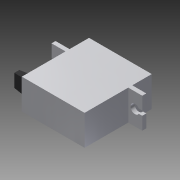
# Autodesk Inventor part: serwo HK15148
Saved by Autodesk Inventor 2013 (Build 170138000, 138)
## iProperties
Created: 2013-03-06
Part Number: serwo HK15148
Material: Generic
Document SubType Name: Modeling
Designer: Masta
Density: 1 g/cm^3
Author: Masta
Autodesk Inventor part; units mm, degrees
ref_plane "YZ Plane" through (0, 0, 0) normal (1, 0, 0) x (0, 1, 0)
ref_plane "XZ Plane" through (0, 0, 0) normal (0, 1, 0) x (-1, 0, 0)
ref_plane "XY Plane" through (0, 0, 0) normal (0, 0, 1) x (1, 0, 0)
sketch "Sketch1" plane through (0, 0, 0) normal (0, 1, 0) x (-1, 0, 0)
  line L0 (14, 6.75) -> (-14, 6.75)
  line L1 (-14, 6.75) -> (-14, -6.75)
  line L2 (-14, -6.75) -> (14, -6.75)
  line L3 (14, -6.75) -> (14, 6.75)
  line L4 (14, 6.75) -> (-14, -6.75) construction
  line L5 (-14, 6.75) -> (14, -6.75) construction
  line L6 (20.25, -6.75) -> (20.25, -1)
  line L7 (14, -6.75) -> (20.25, -6.75)
  line L8 (14, 6.75) -> (20.25, 6.75)
  line L9 (-14, 6.75) -> (-20.25, 6.75)
  line L10 (-14, -6.75) -> (-20.25, -6.75)
  line L11 (-14, 0) -> (14, 0) construction
  line L12 (0, 6.75) -> (0, -6.75) construction
  line L13 (20.25, -1) -> (18.7321, -1)
  line L14 (20.25, 1) -> (18.7321, 1)
  circle A0 centre (17, 0) radius 2
  line L15 (-20.25, 6.75) -> (-20.25, -6.75)
  line L16 (20.25, 1) -> (20.25, 6.75)
  line L17 (20.25, -1) -> (20.25, 1)
  line L18 (-20.25, 6.75) -> (20.25, -6.75) construction
  line L19 (-20.25, -6.75) -> (20.25, 6.75) construction
  line L20 (17, 0) -> (14, 0) construction
  point P0 (0, 0)
  point P1 (0, 0)
  dimension "d0" = 28
  dimension "d1" = 13.5
  dimension "d2" = 40.5
  dimension "d40" = 4
  dimension "d41" = 2
  dimension "d42" = 17
  constraints: 42 end point, 7 midpoint, 7 parallel, 5 perpendicular, 2 collinear, 2 point on circle, 1 centre point, 1 coincident, 1 horizontal, 1 other
  measures "d0" distance of L2.end L1.end
  measures "d1" distance of L1.end L0.end
  measures "d2" distance of L10.end L6.start
  measures "d40" diameter of A0
  measures "d41" distance between parallel lines of L14 L13
  measures "d42" distance of point (0, 0) L20.start
extrude "Extrusion1" add sketch "Sketch1" along normal blind 10.5 and the other way blind 19.5 contours L3 L2 L1 L0
extrude "Extrusion2" add sketch "Sketch1" along normal blind 1.8 contours L8 L16 L14 A0 L13 L6 L7 L3
sketch "Sketch2" plane through (0, 10.5, 0) normal (0, 1, 0) x (1, 0, 0)
  line L0 (-14, 6.75) -> (-14, -6.75) projected
  circle A0 centre (-4, 0) radius 6.5
  line L1 (-4, 0) -> (0, 0) construction
  dimension "d14" = 13
  dimension "d15" = 10
  constraints: 2 end point, 1 centre point, 1 perpendicular
  measures "d14" diameter of A0
  measures "d15" distance from line of L1.start L0
extrude "Extrusion3" add sketch "Sketch2" along normal blind 0.1
sketch "Sketch3" plane through (-4, 10.6, 0) normal (0, 1, 0) x (1, 0, 0)
  circle A0 centre (0, 0) radius 6.5 projected
  circle A1 centre (0, 0) radius 3
  point P0 (4, 0)
  dimension "d18" = 6
  constraints: 1 centre point, 1 coincident
  measures "d18" diameter of A1
extrude "Extrusion4" add sketch "Sketch3" along normal blind 3.5 contours A1
sketch "Sketch4" plane through (-14, -19.5, -6.75) normal (-1, 0, 0) x (0, 0, 1)
  line L0 (13.5, 19.5) -> (0, 19.5) projected
  line L1 (3.25, 3) -> (10.25, 3)
  line L2 (10.25, 3) -> (10.25, 6.5)
  line L3 (10.25, 6.5) -> (3.25, 6.5)
  line L4 (3.25, 6.5) -> (3.25, 3)
  line L5 (3.25, 3) -> (10.25, 6.5) construction
  line L6 (10.25, 3) -> (3.25, 6.5) construction
  line L7 (6.75, 19.5) -> (6.75, 4.75) construction
  dimension "d21" = 7
  dimension "d22" = 3.5
  dimension "d23" = 13
  constraints: 14 end point, 3 parallel, 2 midpoint, 1 horizontal, 1 perpendicular
  measures "d21" distance of L3.end L2.end
  measures "d22" distance of L2.end L1.end
  measures "d23" distance between parallel lines of L0 L3
extrude "Extrusion5" add sketch "Sketch4" along normal blind 7 draft -5
sketch "Sketch6" plane through (0, 10.5, 0) normal (0, 1, 0) x (1, 0, 0)
  line L0 (9.5237, -5.9702) -> (9.5237, 8.1574) construction
  line L1 (9.5237, 8.1574) -> (13.0974, 8.1574) construction
  line L2 (13.0974, 8.1574) -> (13.0974, -5.9702) construction
  line L3 (13.0974, -5.9702) -> (9.5237, -5.9702) construction
  line L4 (11.569, -4.3154) -> (11.569, -4.5812)
  line L5 (11.569, -4.5812) -> (10.5901, -4.5812)
  line L6 (10.5901, -4.5812) -> (10.5901, -5.5018)
  line L7 (10.5901, -5.5018) -> (11.569, -5.5018)
  line L8 (11.569, -5.5018) -> (11.569, -5.7676)
  line L9 (11.569, -5.7676) -> (9.569, -5.7676)
  line L10 (9.569, -5.7676) -> (9.569, -5.5018)
  line L11 (9.569, -5.5018) -> (10.3535, -5.5018)
  line L12 (10.3535, -5.5018) -> (10.3535, -4.5812)
  line L13 (10.3535, -4.5812) -> (9.569, -4.5812)
  line L14 (9.569, -4.5812) -> (9.569, -4.3154)
  line L15 (9.569, -4.3154) -> (11.569, -4.3154)
  line L16 (11.569, -2.4516) -> (11.569, -2.7968)
  line L17 (11.569, -2.7968) -> (10.6387, -3.5278)
  line L18 (10.6387, -3.5278) -> (10.77, -3.6445)
  line L19 (10.77, -3.6445) -> (11.569, -3.6445)
  line L20 (11.569, -3.6445) -> (11.569, -3.9103)
  line L21 (11.569, -3.9103) -> (9.569, -3.9103)
  line L22 (9.569, -3.9103) -> (9.569, -3.6445)
  line L23 (9.569, -3.6445) -> (10.488, -3.6445)
  line L24 (10.488, -3.6445) -> (9.569, -2.8244)
  line L25 (9.569, -2.8244) -> (9.569, -2.5002)
  line L26 (9.569, -2.5002) -> (10.4621, -3.3284)
  line L27 (10.4621, -3.3284) -> (11.569, -2.4516)
  line L28 (11.569, -1.2166) -> (11.569, -2.1923)
  line L29 (11.569, -2.1923) -> (11.3648, -2.1923)
  line L30 (11.3648, -2.1923) -> (11.3648, -1.8292)
  line L31 (11.3648, -1.8292) -> (10.0245, -1.8292)
  line L32 (10.0245, -1.8292) -> (10.0245, -2.1923)
  line L33 (10.0245, -2.1923) -> (9.8413, -2.1923)
  spline S0 degree 2 poles (9.8413, -2.1923) (9.8413, -1.9864) (9.7246, -1.7919) (9.5626, -1.779) knots 0 0 0 1 2 2 2
  line L34 (9.5626, -1.779) -> (9.5626, -1.5715)
  line L35 (9.5626, -1.5715) -> (11.3648, -1.5715)
  line L36 (11.3648, -1.5715) -> (11.3648, -1.2166)
  line L37 (11.3648, -1.2166) -> (11.569, -1.2166)
  spline S1 degree 2 poles (10.9337, 0.3636) (11.078, 0.3636) (11.3243, 0.2713) (11.4151, 0.187) knots 0 0 0 1 2 2 2
  spline S2 degree 2 poles (11.4151, 0.187) (11.5058, 0.1027) (11.6112, -0.1485) (11.6112, -0.3041) knots 0 0 0 1 2 2 2
  spline S3 degree 2 poles (11.6112, -0.3041) (11.6112, -0.4467) (11.548, -0.7255) (11.4977, -0.8276) knots 0 0 0 1 2 2 2
  line L38 (11.4977, -0.8276) -> (11.2141, -0.8276)
  line L39 (11.2141, -0.8276) -> (11.2141, -0.8081)
  spline S4 degree 2 poles (11.2141, -0.8081) (11.2368, -0.7774) (11.2951, -0.6623) (11.3211, -0.5926) knots 0 0 0 1 2 2 2
  spline S5 degree 2 poles (11.3211, -0.5926) (11.3486, -0.5132) (11.3794, -0.3819) (11.3794, -0.2992) knots 0 0 0 1 2 2 2
  spline S6 degree 2 poles (11.3794, -0.2992) (11.3794, -0.2182) (11.3211, -0.0658) (11.2579, -0.0107) knots 0 0 0 1 2 2 2
  spline S7 degree 2 poles (11.2579, -0.0107) (11.1979, 0.0395) (11.0391, 0.0914) (10.9321, 0.0914) knots 0 0 0 1 2 2 2
  spline S8 degree 2 poles (10.9321, 0.0914) (10.8251, 0.0914) (10.689, 0.033) (10.6436, -0.0221) knots 0 0 0 1 2 2 2
  spline S9 degree 2 poles (10.6436, -0.0221) (10.5934, -0.0788) (10.5512, -0.2474) (10.5512, -0.3495) knots 0 0 0 1 2 2 2
  spline S10 degree 2 poles (10.5512, -0.3495) (10.5512, -0.4597) (10.5853, -0.6785) (10.5998, -0.7449) knots 0 0 0 1 2 2 2
  line L40 (10.5998, -0.7449) -> (9.569, -0.7449)
  line L41 (9.569, -0.7449) -> (9.569, 0.3523)
  line L42 (9.569, 0.3523) -> (9.8041, 0.3523)
  line L43 (9.8041, 0.3523) -> (9.8041, -0.4872)
  line L44 (9.8041, -0.4872) -> (10.3373, -0.4872)
  spline S11 degree 2 poles (10.3373, -0.4872) (10.3308, -0.4386) (10.3259, -0.3446) (10.3259, -0.3057) knots 0 0 0 1 2 2 2
  spline S12 degree 2 poles (10.3259, -0.3057) (10.3259, -0.1517) (10.3762, 0.0606) (10.4507, 0.1578) knots 0 0 0 1 2 2 2
  spline S13 degree 2 poles (10.4507, 0.1578) (10.5253, 0.2567) (10.7522, 0.3636) (10.9337, 0.3636) knots 0 0 0 1 2 2 2
  line L45 (11.569, 1.785) -> (11.569, 0.8094)
  line L46 (11.569, 0.8094) -> (11.3648, 0.8094)
  line L47 (11.3648, 0.8094) -> (11.3648, 1.1724)
  line L48 (11.3648, 1.1724) -> (10.0245, 1.1724)
  line L49 (10.0245, 1.1724) -> (10.0245, 0.8094)
  line L50 (10.0245, 0.8094) -> (9.8413, 0.8094)
  spline S14 degree 2 poles (9.8413, 0.8094) (9.8413, 1.0152) (9.7246, 1.2097) (9.5626, 1.2226) knots 0 0 0 1 2 2 2
  line L51 (9.5626, 1.2226) -> (9.5626, 1.4301)
  line L52 (9.5626, 1.4301) -> (11.3648, 1.4301)
  line L53 (11.3648, 1.4301) -> (11.3648, 1.785)
  line L54 (11.3648, 1.785) -> (11.569, 1.785)
  line L55 (10.8818, 3.4398) -> (10.8818, 3.2016)
  line L56 (10.8818, 3.2016) -> (11.569, 3.2016)
  line L57 (11.569, 3.2016) -> (11.569, 2.9439)
  line L58 (11.569, 2.9439) -> (10.8818, 2.9439)
  line L59 (10.8818, 2.9439) -> (10.8818, 2.0606)
  line L60 (10.8818, 2.0606) -> (10.5998, 2.0606)
  line L61 (10.5998, 2.0606) -> (9.569, 2.9552)
  line L62 (9.569, 2.9552) -> (9.569, 3.2016)
  line L63 (9.569, 3.2016) -> (10.6663, 3.2016)
  line L64 (10.6663, 3.2016) -> (10.6663, 3.4398)
  line L65 (10.6663, 3.4398) -> (10.8818, 3.4398)
  line L66 (10.6663, 2.9439) -> (9.8851, 2.9439)
  line L67 (9.8851, 2.9439) -> (10.6663, 2.2713)
  line L68 (10.6663, 2.2713) -> (10.6663, 2.9439)
  spline S15 degree 2 poles (11.6144, 4.2583) (11.6144, 4.1092) (11.5253, 3.8645) (11.4426, 3.7786) knots 0 0 0 1 2 2 2
  spline S16 degree 2 poles (11.4426, 3.7786) (11.3616, 3.6943) (11.1412, 3.6068) (11.0164, 3.6068) knots 0 0 0 1 2 2 2
  spline S17 degree 2 poles (11.0164, 3.6068) (10.8543, 3.6068) (10.582, 3.7802) (10.501, 3.9455) knots 0 0 0 1 2 2 2
  line L69 (10.501, 3.9455) -> (10.4929, 3.9455)
  spline S18 degree 2 poles (10.4929, 3.9455) (10.407, 3.798) (10.2028, 3.6554) (10.0504, 3.6554) knots 0 0 0 1 2 2 2
  spline S19 degree 2 poles (10.0504, 3.6554) (9.8251, 3.6554) (9.5237, 3.9957) (9.5237, 4.2583) knots 0 0 0 1 2 2 2
  spline S20 degree 2 poles (9.5237, 4.2583) (9.5237, 4.5306) (9.8089, 4.8596) (10.0326, 4.8596) knots 0 0 0 1 2 2 2
  spline S21 degree 2 poles (10.0326, 4.8596) (10.1671, 4.8596) (10.4297, 4.7024) (10.5042, 4.5549) knots 0 0 0 1 2 2 2
  line L70 (10.5042, 4.5549) -> (10.5123, 4.5549)
  spline S22 degree 2 poles (10.5123, 4.5549) (10.5934, 4.7299) (10.8267, 4.9098) (11.0115, 4.9098) knots 0 0 0 1 2 2 2
  spline S23 degree 2 poles (11.0115, 4.9098) (11.2676, 4.9098) (11.6144, 4.5371) (11.6144, 4.2583) knots 0 0 0 1 2 2 2
  spline S24 degree 2 poles (11.0374, 4.6343) (10.9143, 4.6343) (10.7684, 4.5371) (10.6938, 4.3993) knots 0 0 0 1 2 2 2
  spline S25 degree 2 poles (10.6938, 4.3993) (10.6679, 4.3539) (10.6079, 4.2016) (10.569, 4.106) knots 0 0 0 1 2 2 2
  spline S26 degree 2 poles (10.569, 4.106) (10.642, 3.9957) (10.8592, 3.8774) (10.9969, 3.8774) knots 0 0 0 1 2 2 2
  spline S27 degree 2 poles (10.9969, 3.8774) (11.1784, 3.8774) (11.4151, 4.0962) (11.4151, 4.2615) knots 0 0 0 1 2 2 2
  spline S28 degree 2 poles (11.4151, 4.2615) (11.4151, 4.4301) (11.2125, 4.6343) (11.0374, 4.6343) knots 0 0 0 1 2 2 2
  spline S29 degree 2 poles (10.0358, 4.597) (9.9013, 4.597) (9.7214, 4.4171) (9.7214, 4.2567) knots 0 0 0 1 2 2 2
  spline S30 degree 2 poles (9.7214, 4.2567) (9.7214, 4.1108) (9.8818, 3.9244) (10.0196, 3.9244) knots 0 0 0 1 2 2 2
  spline S31 degree 2 poles (10.0196, 3.9244) (10.1185, 3.9244) (10.2562, 4.0201) (10.3113, 4.1157) knots 0 0 0 1 2 2 2
  spline S32 degree 2 poles (10.3113, 4.1157) (10.334, 4.1562) (10.4135, 4.328) (10.4361, 4.3977) knots 0 0 0 1 2 2 2
  spline S33 degree 2 poles (10.4361, 4.3977) (10.347, 4.5144) (10.1574, 4.597) (10.0358, 4.597) knots 0 0 0 1 2 2 2
  point P0 (0, 0)
  constraints: 2 other
emboss "Emboss1" sketch "Sketch6" operation cut depth 0.1 direction (0, -1, 0)
hole "Hole1" at (-4, 14.1, 0) direction (0, -1, 0) diameter 2.459 depth 8 tip angle 118 thread size "M3x0.5" class "6H" standard "ISO Metric profile"
mirror "Mirror1" about plane through (0, 0, 0) normal (1, 0, 0) of "Extrusion2"
body "Solid1"
